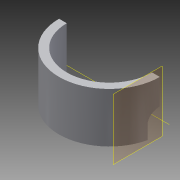
# Autodesk Inventor part: BurkolatPVCszenzorFedel
Saved by Autodesk Inventor 2015 SP1 (Build 190203100, 203)
## iProperties
Created: 2014-11-14
Part Number: BurkolatPVCszenzorFedel
Material: PVC-Piping
Document SubType Name: Modeling
Designer: laca
Density: 1.4 g/cm^3
Appearance: Smooth - White
Mass: 56.2258 g
Surface Area: 139.252 cm^2
Volume: 40.1613 cm^3
Author: laca
Autodesk Inventor part; units mm, degrees
ref_plane "YZ Plane" through (0, 0, 0) normal (1, 0, 0) x (0, 1, 0)
ref_plane "XZ Plane" through (0, 0, 0) normal (0, 1, 0) x (-1, 0, 0)
ref_plane "XY Plane" through (0, 0, 0) normal (0, 0, 1) x (1, 0, 0)
sketch "Sketch1" plane through (0, 0, 0) normal (0, 1, 0) x (-1, 0, 0)
  circle A0 centre (0, 0) radius 45.5
  circle A1 centre (0, 0) radius 38.5
  line L0 (-45.5, 0) -> (-38.5, 0)
  line L1 (38.5, 0) -> (45.5, 0)
  dimension "d1" = 7
  dimension "d4" = 91
  constraints: 4 end point, 4 point on circle, 2 centre point, 2 coincident, 2 horizontal
  measures "d1" radial gap between concentric circles of A0 A1
  measures "d4" diameter of A0
extrude "Extrusion1" add sketch "Sketch1" along normal blind 45 contours L1 A1 L0 A0 picked at (-42.8352, 3.1533)
ref_plane "Work Plane1" through (45.5, 0, 0) normal (1, 0, 0) x (0, 1, 0)
sketch "Sketch2" plane through (45.5, 0, 0) normal (1, 0, 0) x (0, 1, 0)
  arc A0 (22, 0) -> (12, 10) centre (12, 0) ccw
  line L0 (0, 0) -> (0, 45.5) projected
  line L1 (0, 0) -> (45, 0) projected
  line L2 (22, 0) -> (22, 0)
  line L3 (0, 0) -> (45, 0) projected
  line L4 (2, 0) -> (2, 0)
  line L5 (22, 0) -> (2, 0)
  line L6 (12, 10) -> (0, 10)
  line L7 (0, 38.5) -> (0, 0) projected
  line L8 (0, 10) -> (0, 0)
  line L9 (0, 0) -> (12, 0)
  dimension "d7" = 20
  dimension "KisFogaskerekBesulyesztese" = 12
  dimension "d9" = 0
  constraints: 12 end point, 3 point on line, 2 perpendicular, 2 point on circle, 1 centre point, 1 collinear, 1 parallel, 1 tangent, 1 vertical
  measures "d7" diameter of A0
  measures "KisFogaskerekBesulyesztese" distance from line of L9.end L0
  measures "d9" distance from line of L1 L9.end
extrude "Extrusion2" cut sketch "Sketch2" against normal blind 50
equation "\"d1\" = PVCfalVastagsag"
equation "\"d4\" = KulsoAtmeroPVCcso"
equation "\"KisFogaskerekBesulyesztese\" = KisFogaskerekBesulyesztes"
equation "\"PVCfalVastagsag\" = 7"
equation "\"KulsoAtmeroPVCcso\" = 91"
equation "\"KisFogaskerekBesulyesztes\" = 12"
body "Solid2"
